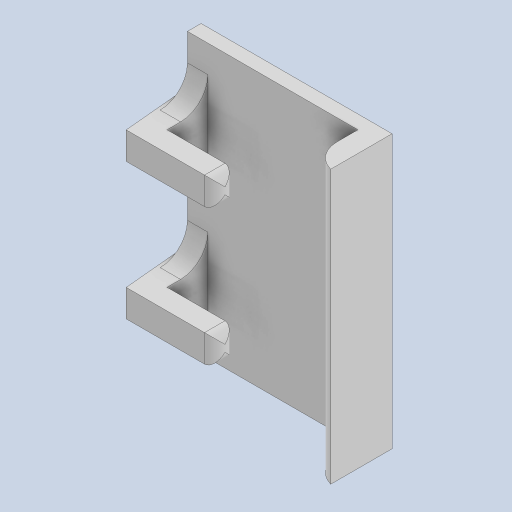
# Autodesk Inventor part: Supporto anello
Saved by Autodesk Inventor 2023.2 (Build 272271030, 271C)
## iProperties
Created: 2022-12-03
Part Number: Supporto anello
Material: Generico
Document SubType Name: Modeling
Designer: daler
Density: 1 g/cm^3
Appearance: Default
Author: daler
Autodesk Inventor part; units mm, degrees
ref_plane "YZ Plane" through (0, 0, 0) normal (1, 0, 0) x (0, 1, 0)
ref_plane "XZ Plane" through (0, 0, 0) normal (0, 1, 0) x (-1, 0, 0)
ref_plane "XY Plane" through (0, 0, 0) normal (0, 0, 1) x (1, 0, 0)
sketch "Schizzo1" plane through (0, 0, 0) normal (0, 0, 1) x (1, 0, 0)
  line L0 (-7, 10) -> (7, 10)
  line L1 (7, 10) -> (7, -10)
  line L2 (7, -10) -> (-7, -10)
  line L3 (-7, -10) -> (-7, 10)
  line L4 (-7, 10) -> (7, -10) construction
  line L5 (7, 10) -> (-7, -10) construction
  line L6 (-5.5, 10) -> (-5.5, -10)
  line L7 (5.5, 10) -> (5.5, -10)
  line L8 (-7, 6) -> (-5.5, 6)
  line L9 (-7, 4) -> (-5.5, 4)
  line L10 (-7, -4) -> (-5.5, -4)
  line L11 (-7, -6) -> (-5.5, -6)
  line L12 (-7, 6) -> (-7.5, 6)
  line L13 (-7.5, 6) -> (-7.5, 4)
  line L14 (-7.5, 4) -> (-7, 4)
  line L15 (-7, 4) -> (-7, 6)
  line L16 (-7, -4) -> (-7.5, -4)
  line L17 (-7.5, -4) -> (-7.5, -6)
  line L18 (-7.5, -6) -> (-7, -6)
  line L19 (-7, -6) -> (-7, -4)
  point P0 (0, 0)
  point P1 (0, 0)
  point P2 (-6.25, 4)
  point P3 (-6.25, -6)
  point P4 (-7, 5)
  dimension "d0" = 14
  dimension "d1" = 20
  dimension "d2" = 1.5
  dimension "d3" = 1.5
  dimension "d4" = 4
  dimension "d5" = 2
  dimension "d6" = 2
  dimension "d7" = 4
  dimension "d19" = 0.5
  constraints: 40 end point, 13 point on line, 9 perpendicular, 6 parallel, 4 midpoint, 3 horizontal, 1 coincident
  measures "d0" distance of L0.start L0.end
  measures "d1" distance of L0.end L1.end
  measures "d2" distance between parallel lines of L3 L6
  measures "d3" distance between parallel lines of L1 L7
  measures "d4" distance between parallel lines of L0 L8
  measures "d5" distance from line of point (-6.25, 4) L8
  measures "d6" distance from line of point (-6.25, -6) L10
  measures "d7" distance between parallel lines of L2 L11
  measures "d19" distance from line of L13 point (-7, 5)
extrude "Estrusione1" add sketch "Schizzo1" along normal blind 1 contours L0 L6 L8 L3 | L0 L7 L2 L6 | L8 L6 L9 L3 | L0 L1 L2 L7 | L9 L6 L10 L3 | L10 L6 L11 L3 | L2 L3 L11 L6
extrude "Estrusione2" add sketch "Schizzo1" along normal blind 4.5 contours L0 L1 L2 L7
extrude "Estrusione3" add sketch "Schizzo1" along normal blind 5.5 contours L8 L6 L9 L3 | L10 L6 L11 L3
sketch "Schizzo2" plane through (-5.5, 4, 1) normal (1, 0, 0) x (0, 0, -1)
  line L0 (0, -10) -> (-4.5, -10) projected
  line L1 (-3, -10) -> (-3, -8)
  line L2 (0, -8) -> (-4.5, -8) projected
  line L3 (0, 0) -> (-4.5, 0) projected
  line L4 (-3, 0) -> (-3, 2)
  line L5 (0, 2) -> (-4.5, 2) projected
  line L6 (-4.5, -10) -> (-4.5, -8) projected
  line L7 (-3, 0) -> (-4.5, 0)
  line L8 (-4.5, 0) -> (-4.5, 2) projected
  line L9 (-4.5, 2) -> (-3, 2)
  point P0 (1, -4)
  dimension "d14" = 1.5
  constraints: 8 end point, 6 point on line, 1 horizontal, 1 parallel, 1 vertical
  measures "d14" distance between parallel lines of L1 L6
extrude "Estrusione4" add sketch "Schizzo2" along normal blind 5
fillet "Raccordo1" radius 2 5 edges at (-6.25, -6, 1) (-6.25, -4, 1) (-6.25, 4, 1) (-6.25, 6, 1) (5.5, 0, 4.5)
fillet "Raccordo2" radius 0.75 8 edges at (-0.5, 5, 5.5) (-0.5, 5, 4) (-0.5, -5, 5.5) (-0.5, -5, 4) (-0.5, -6, 4.75) (-0.5, -4, 4.75) (-0.5, 4, 4.75) (-0.5, 6, 4.75)
extrude "Estrusione5" add sketch "Schizzo1" along normal blind 5.5 contours L3 L14 L13 L12 | L3 L18 L17 L16
sketch "Schizzo3" plane through (-7, -6, 3) normal (0, -1, 0) x (1, 0, 0)
  line L0 (-0.5, 2.5) -> (5.75, 2.5) projected
  line L1 (0.0105, 2.5) -> (-0.5, 2.5)
  line L2 (-0.5, 2.5) -> (-0.5, -3)
  line L3 (-0.5, -3) -> (0.0105, 2.5)
  point P0 (7, -3)
  point P1 (0.0105, 2.5)
  constraints: 6 end point, 1 horizontal, 1 perpendicular
extrude "Estrusione6" cut sketch "Schizzo3" against normal blind 90
fillet "Raccordo3" radius 0.5 1 edges at (-7.5, 5, 0)
equation "\"d0\" = Larghezza"
equation "\"d1\" = Lunghezza"
equation "\"d2\" = Parete"
equation "\"d3\" = d2"
equation "\"d4\" = Gancio_bordo"
equation "\"d5\" = Gancio_larghezza_base"
equation "\"d6\" = d5"
equation "\"d7\" = d4"
equation "\"Lunghezza\" = 20"
equation "\"Larghezza\" = 14"
equation "\"Parete\" = 1.5"
equation "\"Gancio_gancio\" = 8"
equation "\"Gancio_bordo\" = 4"
equation "\"Gancio_larghezza_base\" = 2"
equation "\"Gancio_spessore\" = 1"
equation "\"Gancio_altezza\" = 5.5"
equation "\"Altezza_parete\" = 4.5"
equation "\"Spessore_base\" = 1"
equation "\"Gancio_larghezza\" = 1.5"
equation "\"Gancio_estrusione\" = 5"
